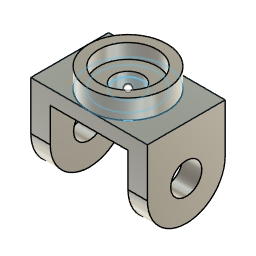
3d_shape1 (Autodesk Fusion 360 design; units mm, degrees)
Autodesk Fusion 360 part; units mm, degrees
sketch "Sketch1" plane through (0, 0, 0) normal (1, 0, 0) x (0, 1, 0)
  line L0 (0, 0) -> (80, 0)
  line L1 (80, 0) -> (80, -50)
  line L2 (80, -50) -> (0, -50)
  line L3 (0, -50) -> (0, 0)
  arc A0 (0, -50) -> (80, -50) centre (40, -50) ccw
  circle A1 centre (40, -50) radius 16
  constraint horizontal L0
  constraint vertical L1
  constraint horizontal L2
  constraint vertical L3
  constraint coincident L0.start L3.end
  constraint midpoint L2 A0.centre
  constraint concentric A0 A1
sketch "Sketch2" plane through (0, 0, 0) normal (1, 0, 0) x (0, 1, 0)
extrude "Extrude1" add sketch "Sketch1" along normal blind 120 contours L0 L1 L2 L3 A1 | L2 A0 A1
sketch "Sketch3" plane through (0, 0, 0) normal (1, 0, 0) x (0, 1, 0)
sketch "Sketch4" plane through (0, 0, 0) normal (0, -1, 0) x (1, 0, 0)
  line L0 (0, 0) -> (0, -50)
  line L1 (0, -50) -> (120, -50)
  line L2 (120, -50) -> (120, 0)
  line L3 (120, 0) -> (0, 0)
  line L4 (0, 0) -> (20, 0)
  line L5 (0, 0) -> (0, -15)
  line L6 (20, -14.9206) -> (100, -14.9206)
  line L7 (100, -14.9206) -> (100, -90)
  line L8 (100, -90) -> (20, -90)
  line L9 (20, -90) -> (20, -14.9206)
  dimension "d3" = 20
  dimension "d4" = 15
  constraint coincident L0.start L3.end
  constraint perpendicular L0 L4
  constraint perpendicular L3 L5
  constraint horizontal L6
  constraint vertical L7
  constraint horizontal L8
  constraint vertical L9
  measures "d3" distance of L0.start L4.end
  measures "d4" distance of L0.start L5.end
extrude "Extrude2" cut sketch "Sketch4" against normal blind 90 contours L1 L6 L7 L9 | L1 L7 L8 L9
sketch "Sketch5" plane through (0, 0, 0) normal (0, 0, 1) x (-1, 0, 0)
  line L0 (0, -80) -> (0, 0)
  line L1 (0, 0) -> (-120, 0)
  line L2 (-120, 0) -> (-120, -80)
  line L3 (-120, -80) -> (0, -80)
sketch "Sketch6" plane through (0, 0, 0) normal (0, 0, 1) x (-1, 0, 0)
  circle A0 centre (-60, -40) radius 40
  circle A1 centre (-60, -40) radius 30
  circle A2 centre (-60, -40) radius 15
  dimension "d7" = 60
  dimension "d8" = 30
  constraint concentric A0 A1
  constraint concentric A0 A2
  measures "d7" diameter of A1
  measures "d8" diameter of A2
extrude "Extrude4" cut sketch "Sketch6" against normal blind 25 contours A2
extrude "Extrude5" add sketch "Sketch6" along normal blind 5 contours A1
extrude "Extrude6" add sketch "Sketch6" along normal blind 20 contours A0
extrude "Extrude3" [suppressed]
sketch "Sketch7" plane through (0, 0, 0) normal (0, 0, 1) x (-1, 0, 0)
